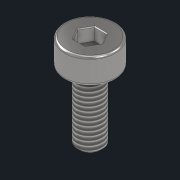
# Autodesk Inventor part: M3-8
Saved by Autodesk Inventor 2021 (Build 250183000, 183)
## iProperties
Created: 2021-06-08
Part Number: M3-8
Material: Steel, Carbon
Document SubType Name: Modeling
Designer: arbra
Density: 7.85 g/cm^3
Appearance: Semi-Polished
Author: arbra
Autodesk Inventor part; units mm, degrees
ref_plane "YZ Plane" through (0, 0, 0) normal (1, 0, 0) x (0, 1, 0)
ref_plane "XZ Plane" through (0, 0, 0) normal (0, 1, 0) x (-1, 0, 0)
ref_plane "XY Plane" through (0, 0, 0) normal (0, 0, 1) x (1, 0, 0)
sketch "Sketch1" plane through (0, 0, 0) normal (0, 1, 0) x (-1, 0, 0)
  circle A0 centre (0, 0) radius 3
  dimension "d0" = 6
  constraints: 1 centre point, 1 coincident
  measures "d0" diameter of A0
extrude "Extrusion1" add sketch "Sketch1" against normal blind 3
sketch "Sketch2" plane through (0, -3, 0) normal (0, -1, 0) x (1, 0, 0)
  circle A0 centre (0, 0) radius 1.5
  dimension "d3" = 3
  constraints: 1 centre point, 1 coincident
  measures "d3" diameter of A0
extrude "Extrusion2" add sketch "Sketch2" along normal blind 8
sketch "Sketch3" plane through (0, 0, 0) normal (0, 1, 0) x (1, 0, 0)
  circle A0 centre (0, 0) radius 1.5 construction
  line L0 (1.4434, 0) -> (0.7217, -1.25)
  line L1 (0.7217, -1.25) -> (-0.7217, -1.25)
  line L2 (-0.7217, -1.25) -> (-1.4434, 0)
  line L3 (-1.4434, 0) -> (-0.7217, 1.25)
  line L4 (-0.7217, 1.25) -> (0.7217, 1.25)
  line L5 (0.7217, 1.25) -> (1.4434, 0)
  dimension "d8" = 2.5
  constraints: 12 end point, 1 coincident, 1 horizontal, 13 other
  measures "d8" distance between parallel lines of L1 L4
extrude "Extrusion3" cut sketch "Sketch3" against normal blind 1.5
chamfer "Chamfer1" distance 0.25 angle 45 1 edges at (-1.5, -11, 0)
fillet "Fillet1" radius 0.25 2 edges at (3, 0, 0) (3, -3, 0)
chamfer "Chamfer2" distance 0.1 angle 45 6 edges at (0, 0, -1.25) (1.0825, 0, -0.625) (1.0825, 0, 0.625) (0, 0, 1.25) (-1.0825, 0, 0.625) (-1.0825, 0, -0.625)
thread "Thread2" size "M3x0.5" class "6g" standard "ANSI Metric M Profile" full length
body "Solid1"
